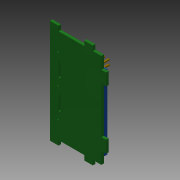
# Autodesk Inventor part: Microcontroller_board_Nano_square
Saved by Autodesk Inventor 2016 (Build 200138000, 138)
## iProperties
Created: 2014-12-25
Part Number: Microcontroller_board_Nano_square
Material: ABS Plastic
Document SubType Name: Modeling
Designer: Openlab
Density: 1.06 g/cm^3
Appearance: Smooth - Dark Forest Green
Mass: 9.08054 g
Surface Area: 59.127 cm^2
Volume: 8.56654 cm^3
Author: Openlab
Autodesk Inventor part; units mm, degrees
ref_plane "YZ Plane" through (0, 0, 0) normal (1, 0, 0) x (0, 1, 0)
ref_plane "XZ Plane" through (0, 0, 0) normal (0, 1, 0) x (-1, 0, 0)
ref_plane "XY Plane" through (0, 0, 0) normal (0, 0, 1) x (1, 0, 0)
sketch "Sketch1" plane through (0, 0, 0) normal (0, 1, 0) x (-1, 0, 0)
  line L0 (15, 17.8107) -> (15, 41.4147) construction
  line L1 (30, 60.5) -> (30, 0)
  line L2 (25, 17.5) -> (25, 26)
  line L3 (25, 26) -> (24, 26)
  line L4 (24, 26) -> (24, 17.5)
  line L5 (24, 17.5) -> (25, 17.5)
  line L6 (24, 34.5) -> (25, 34.5)
  line L7 (25, 34.5) -> (25, 43)
  line L8 (25, 43) -> (24, 43)
  line L9 (24, 43) -> (24, 34.5)
  line L10 (25, 57.75) -> (25, 60.5)
  line L11 (25, 60.5) -> (30, 60.5)
  line L12 (10, 57.75) -> (10, 60.5)
  line L13 (25, 57.75) -> (10, 57.75)
  line L14 (25, 2.75) -> (25, 0)
  line L15 (25, 0) -> (30, 0)
  line L16 (10, 2.75) -> (10, 0)
  line L17 (25, 2.75) -> (10, 2.75)
  line L18 (0, 50.75) -> (-2.75, 50.75)
  line L19 (-2.75, 50.75) -> (-2.75, 43.75)
  line L20 (-2.75, 43.75) -> (0, 43.75)
  line L21 (0, 16.75) -> (-2.75, 16.75)
  line L22 (-2.75, 16.75) -> (-2.75, 9.75)
  line L23 (-2.75, 9.75) -> (0, 9.75)
  line L24 (17.3275, 30.25) -> (11.5049, 30.25) construction
  line L25 (0, 50.75) -> (0, 57.75)
  line L26 (0, 2.75) -> (0, 9.75)
  line L27 (0, 16.75) -> (0, 43.75)
  line L28 (10, 0) -> (5, 0)
  line L29 (5, 0) -> (5, 2.75)
  line L30 (5, 2.75) -> (0, 2.75)
  line L31 (10, 60.5) -> (5, 60.5)
  line L32 (5, 60.5) -> (5, 57.75)
  line L33 (5, 57.75) -> (0, 57.75)
  point P0 (0, 0)
  point P1 (0, 0)
  point P2 (0, 0)
  point P3 (0, 0)
  point P4 (0, 0)
  point P5 (25.5, 47.25)
  point P6 (25.5, 30.25)
  point P7 (25.5, 13.25)
  dimension "d151" = 8.5
  dimension "d153" = 1
  dimension "d155" = 5
  dimension "d159" = 17
  dimension "d160" = 17
  dimension "d161" = 4.25
  dimension "d162" = 4.25
  dimension "d176" = 4.5
  dimension "d177" = 5
  dimension "d179" = 55
  dimension "d180" = 2.75
  dimension "d182" = 7
  dimension "d183" = 7
  dimension "d184" = 30
  constraints: 68 end point, 19 perpendicular, 12 equal length, 7 horizontal, 5 collinear, 5 point on line, 4 coincident, 4 vertical, 2 parallel, 2 vertical alignment, 3 other
  measures "d151" distance of L8.end L6.start
  measures "d153" distance of L7.end L8.end
  measures "d155" distance between parallel lines of L1 L7
  measures "d159" distance of point (25.5, 30.25) point (25.5, 47.25)
  measures "d160" distance of point (25.5, 13.25) point (25.5, 30.25)
  measures "d161" distance from line of L8 point (25.5, 47.25)
  measures "d162" distance from line of point (25.5, 30.25) L3
  measures "d176" distance from line of L1 point (25.5, 13.25)
  measures "d177" distance of L10.end L1.start
  measures "d179" distance between parallel lines of L17 L13
  measures "d180" distance of L12.start L12.end
  measures "d182" distance between parallel lines of L18 L13
  measures "d183" distance of L18.end L19.end
  measures "d184" distance between parallel lines of L25 L1
extrude "Extrusion1" add sketch "Sketch1" against normal blind 1.5
hole "Hole1" at (-25.5, 0, 47.25) at (-25.5, 0, 30.25) at (-25.5, 0, 13.25) direction (0, -1, 0) diameter 1 end through all
sketch "Sketch4" plane through (0, 0, 0) normal (0, 1, 0) x (1, 0, 0)
  line L0 (-3, -46.55) -> (-3, -3.25)
  line L1 (-3, -3.25) -> (-21, -3.25)
  line L2 (-21, -3.25) -> (-21, -46.55)
  line L3 (-21, -46.55) -> (-3, -46.55)
  line L4 (-25, -2.75) -> (-10, -2.75) projected
  line L5 (-10, -2.75) -> (-25, -2.75) projected
  line L6 (0, -43.75) -> (0, -16.75) projected
  point P0 (0, 0)
  dimension "d188" = 43.3
  dimension "d189" = 18
  dimension "d190" = 3
  dimension "d212" = 0.5
  constraints: 8 end point, 2 vertical, 1 parallel, 1 perpendicular
  measures "d188" distance of L0.start L0.end
  measures "d189" distance of L0.end L1.end
  measures "d190" distance between parallel lines of L6 L0
  measures "d212" distance between parallel lines of L4 L1
extrude "Extrusion11" add sketch "Sketch4" along normal blind 5
sketch "Sketch6" plane through (0, 5, 0) normal (0, 1, 0) x (1, 0, 0)
  line L0 (-17.0504, -18.7342) -> (-12.1007, -13.7844)
  line L1 (-12.1007, -13.7844) -> (-7.1509, -18.7342)
  line L2 (-7.1509, -18.7342) -> (-12.1007, -23.6839)
  line L3 (-12.1007, -23.6839) -> (-17.0504, -18.7342)
  point P0 (0, 0)
  dimension "d198" = 7
  dimension "d199" = 7
  constraints: 8 end point, 2 parallel, 1 perpendicular
  measures "d198" distance of L1.end L2.end
  measures "d199" distance of L0.end L1.end
extrude "Extrusion13" add sketch "Sketch6" along normal blind 2
sketch "Sketch7" plane through (0, 5, 0) normal (0, 1, 0) x (1, 0, 0)
  line L0 (-15.6959, -40.3292) -> (-8.6959, -40.3292)
  line L1 (-8.6959, -40.3292) -> (-8.6959, -45.3292)
  line L2 (-8.6959, -45.3292) -> (-15.6959, -45.3292)
  line L3 (-15.6959, -45.3292) -> (-15.6959, -40.3292)
  point P0 (0, 0)
  dimension "d202" = 7
  dimension "d203" = 5
  constraints: 8 end point, 2 parallel, 1 horizontal, 1 perpendicular
  measures "d202" distance of L1.end L2.end
  measures "d203" distance of L2.end L0.start
extrude "Extrusion14" add sketch "Sketch7" along normal blind 2.5
sketch "Sketch8" plane through (0, 7.5, 0) normal (0, 1, 0) x (1, 0, 0)
  line L0 (-15.3142, -41.2282) -> (-14.6142, -41.2282)
  line L1 (-14.6142, -41.2282) -> (-14.6142, -41.9282)
  line L2 (-14.6142, -41.9282) -> (-15.3142, -41.9282)
  line L3 (-15.3142, -41.9282) -> (-15.3142, -41.2282)
  line L4 (-15.3142, -43.9282) -> (-14.6142, -43.9282)
  line L5 (-14.6142, -43.9282) -> (-14.6142, -44.6282)
  line L6 (-14.6142, -44.6282) -> (-15.3142, -44.6282)
  line L7 (-15.3142, -44.6282) -> (-15.3142, -43.9282)
  line L8 (-12.6142, -41.2282) -> (-11.9142, -41.2282)
  line L9 (-11.9142, -41.2282) -> (-11.9142, -41.9282)
  line L10 (-11.9142, -41.9282) -> (-12.6142, -41.9282)
  line L11 (-12.6142, -41.9282) -> (-12.6142, -41.2282)
  line L12 (-12.6142, -43.9282) -> (-11.9142, -43.9282)
  line L13 (-11.9142, -43.9282) -> (-11.9142, -44.6282)
  line L14 (-11.9142, -44.6282) -> (-12.6142, -44.6282)
  line L15 (-12.6142, -44.6282) -> (-12.6142, -43.9282)
  line L16 (-9.9142, -41.2282) -> (-9.2142, -41.2282)
  line L17 (-9.2142, -41.2282) -> (-9.2142, -41.9282)
  line L18 (-9.2142, -41.9282) -> (-9.9142, -41.9282)
  line L19 (-9.9142, -41.9282) -> (-9.9142, -41.2282)
  line L20 (-9.9142, -43.9282) -> (-9.2142, -43.9282)
  line L21 (-9.2142, -43.9282) -> (-9.2142, -44.6282)
  line L22 (-9.2142, -44.6282) -> (-9.9142, -44.6282)
  line L23 (-9.9142, -44.6282) -> (-9.9142, -43.9282)
  point P0 (0, 0)
  dimension "d206" = 0.7
  dimension "d207" = 2
  dimension "d208" = 2
  dimension "d209" = 2
  constraints: 48 end point, 12 parallel, 10 point on line, 6 equal length, 6 horizontal, 6 perpendicular, 2 collinear
  measures "d206" distance of L0.start L0.end
  measures "d207" distance between parallel lines of L4 L2
  measures "d208" distance between parallel lines of L11 L1
  measures "d209" distance between parallel lines of L19 L9
extrude "Extrusion15" add sketch "Sketch8" along normal blind 5
sketch "Sketch9" plane through (-3, 0, 3.25) normal (0, 0, -1) x (-1, 0, 0)
  line L0 (12.75, 8.5) -> (5.25, 8.5)
  line L1 (5.25, 8.5) -> (5.25, 5)
  line L2 (5.25, 5) -> (12.75, 5)
  line L3 (12.75, 5) -> (12.75, 8.5)
  line L4 (9, 5.7242) -> (9, 7.4058) construction
  line L5 (18, 0) -> (18, 5) projected
  line L6 (0, 5) -> (18, 5) projected
  point P0 (-3, 0)
  dimension "d213" = 7.5
  dimension "d214" = 3.5
  dimension "d215" = 9
  constraints: 10 end point, 2 parallel, 1 collinear, 1 horizontal, 1 perpendicular, 1 vertical, 1 other
  measures "d213" distance of L0.start L0.end
  measures "d214" distance of L2.end L0.start
  measures "d215" distance between parallel lines of L5 L4
extrude "Extrusion16" add sketch "Sketch9" along normal blind 2 and the other way blind 7
sketch "Sketch15" plane through (-3, 0, 1.25) normal (0, 0, -1) x (-1, 0, 0)
  line L0 (12.25, 8.25) -> (5.75, 8.25)
  line L1 (5.75, 8.25) -> (5.75, 5.25)
  line L2 (5.75, 5.25) -> (12.25, 5.25)
  line L3 (12.25, 5.25) -> (12.25, 8.25)
  line L4 (5.25, 8.5) -> (5.25, 5) projected
  line L5 (12.75, 8.5) -> (5.25, 8.5) projected
  point P0 (-3, 0)
  dimension "d242" = 6.5
  dimension "d243" = 3
  dimension "d244" = 0.5
  dimension "d245" = 0.25
  constraints: 8 end point, 2 parallel, 1 horizontal, 1 perpendicular
  measures "d242" distance of L0.start L0.end
  measures "d243" distance of L2.end L0.start
  measures "d244" distance between parallel lines of L4 L1
  measures "d245" distance between parallel lines of L0 L5
extrude "Extrusion20" cut sketch "Sketch15" against normal blind 5
body "Solid1"
